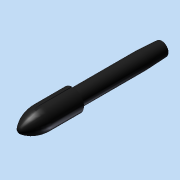
# Autodesk Inventor part: Nib
Saved by Autodesk Inventor 2012 (Build 160160000, 160)
## iProperties
Created: 2015-03-22
Part Number: Nib
Material: Default
Document SubType Name: Modeling
Designer: Jason
Density: 1 g/cm^3
Author: Jason
Autodesk Inventor part; units mm, degrees
ref_plane "YZ Plane" through (0, 0, 0) normal (1, 0, 0) x (0, 1, 0)
ref_plane "XZ Plane" through (0, 0, 0) normal (0, 1, 0) x (-1, 0, 0)
ref_plane "XY Plane" through (0, 0, 0) normal (0, 0, 1) x (1, 0, 0)
sketch "Sketch1" plane through (0, 0, 0) normal (0, 0, 1) x (1, 0, 0)
  point P0 (0, 0)
sketch "Sketch2" plane through (0, 0, 0) normal (1, 0, 0) x (0, 1, 0)
  line L0 (0, 0) -> (0, 27.5)
  line L1 (1.5, 17) -> (1.5, 4)
  line L2 (1.5, 4) -> (1.3, 0)
  line L3 (1.3, 0) -> (0, 0)
  line L4 (1.5, 17) -> (2.1, 17)
  line L5 (2.1, 17) -> (2.1, 23)
  line L6 (1.5, 4) -> (0, 4) construction
  circle A0 centre (0, 26.75) radius 0.75 construction
  arc A1 (2.1, 23) -> (0.5779, 27.228) centre (-4.5333, 23) ccw
  arc A2 (0.5779, 27.228) -> (0, 27.5) centre (0, 26.75) ccw
  line L7 (0, -5.5129) -> (0, 33.0775) projected
  line L8 (2.1, 23) -> (0, 23) construction
  line L9 (-0.75, 26) -> (0.75, 26) construction
  line L10 (0.75, 26) -> (0.75, 27.5) construction
  line L11 (0.75, 27.5) -> (-0.75, 27.5) construction
  line L12 (-0.75, 27.5) -> (-0.75, 26) construction
  dimension "d0" = 27.5
  dimension "d1" = 4
  dimension "d2" = 1.5
  dimension "d3" = 2.1
  dimension "d4" = 1.5
  dimension "d5" = 1.3
  dimension "d6" = 17
  dimension "d8" = 6
  dimension "d15" = 4.5
  constraints: 24 end point, 7 tangent, 6 point on circle, 5 horizontal, 3 centre point, 3 point on line, 3 vertical, 2 parallel, 1 concentric, 1 perpendicular
  measures "d0" distance of L0.start L0.end
  measures "d1" distance between parallel lines of L3 L6
  measures "d2" diameter of A0
  measures "d3" distance from line of L0.start L5
  measures "d4" distance between parallel lines of L0 L1
  measures "d5" distance of L2.end L0.start
  measures "d6" distance between parallel lines of L4 L3
  measures "d8" distance of L4.end L5.end
  measures "d15" distance between parallel lines of L8 L11
revolve "Revolution1" add sketch "Sketch2" angle 360 about axis through (0, 0, -10) along (0, 0, 1)
sketch "Sketch3" plane through (0, 0, 17) normal (0, 0, -1) x (-1, 0, 0)
  circle A0 centre (0, 0) radius 1.5 projected
  circle A1 centre (0, 0) radius 2.1 projected
  line L0 (-0.25, 2.55) -> (0.25, 2.55)
  line L1 (0.25, 2.55) -> (0.25, 1.95)
  line L2 (0.25, 1.95) -> (-0.25, 1.95)
  line L3 (-0.25, 1.95) -> (-0.25, 2.55)
  point P0 (0, 1.95)
  dimension "d10" = 0.15
  dimension "d11" = 0.5
  dimension "d14" = 0.6
  constraints: 8 end point, 2 parallel, 1 horizontal, 1 midpoint, 1 perpendicular, 1 vertical alignment
  measures "d10" distance edge to line of A1 L2
  measures "d11" distance between parallel lines of L1 L3
  measures "d14" distance between parallel lines of L2 L0
extrude "Extrusion1" cut sketch "Sketch3" against normal through all contours L1 L2 L3 A1 | A1 L3 L0 L1 picked at (0.0278, 1.9994)
body "Solid1"
